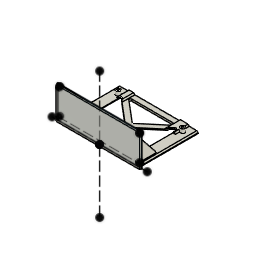
Mainboard Mount - Blank (Autodesk Fusion 360 design; units mm, degrees)
Autodesk Fusion 360 part; units mm, degrees
sketch "Sketch1" plane through (0, 0, 0) normal (0, 1, 0) x (1, 0, 0) in component "Blank Mount"
  line L0 (-75, 0) -> (75, 0) construction
  line L1 (-66, -50) -> (66, -50)
  line L2 (66, -50) -> (66, 0)
  line L3 (66, 0) -> (-66, 0)
  line L4 (-66, 0) -> (-66, -50)
  line L5 (0, -100) -> (0, 100) construction
  circle A0 centre (-63, -47) radius 1.75
  circle A1 centre (-63, -47) radius 3
  circle A2 centre (-63, -6.75) radius 1.75
  circle A3 centre (-63, -6.75) radius 3
  circle A4 centre (63, -47) radius 1.75
  circle A5 centre (63, -47) radius 3
  circle A6 centre (63, -6.75) radius 1.75
  circle A7 centre (63, -6.75) radius 3
  line L6 (-66, -5) -> (66, -5) construction
  dimension "d99_1" = 150
  dimension "d100_1" = 132
  dimension "d101_1" = 50
  dimension "d102_1" = 200
  dimension "d103_1" = 3.5
  dimension "d104_1" = 6
  dimension "d105_1" = 3.5
  dimension "d106_1" = 6
  dimension "d107_1" = 3.5
  dimension "d108_1" = 6
  dimension "d109_1" = 3.5
  dimension "d110_1" = 6
  dimension "d111_1" = 5
  constraint horizontal L0
  constraint midpoint L0 origin
  constraint horizontal L1
  constraint vertical L2
  constraint horizontal L3
  constraint vertical L4
  constraint vertical L5
  constraint midpoint L5 origin
  constraint midpoint L3 origin
  constraint coincident L5 origin
  constraint concentric A0 A1
  constraint concentric A2 A3
  constraint concentric A4 A5
  constraint concentric A6 A7
  constraint horizontal A0.centre A4.centre
  constraint vertical A4.centre A6.centre
  constraint vertical A0.centre A2.centre
  constraint horizontal A2.centre A6.centre
  constraint tangent L1 A1
  constraint tangent L4 A1
  constraint tangent L2 A5
  constraint coincident L4 L6.start
  constraint coincident L2 L6.end
  constraint perpendicular L2 L6
  constraint tangent A6 L6
  measures "d99_1" distance of L0.start L0.end
  measures "d100_1" distance of L1.start L1.end
  measures "d101_1" distance of L1.start L3.end
  measures "d102_1" distance of L5.start L5.end
  measures "d103_1" diameter of A0
  measures "d104_1" diameter of A1
  measures "d105_1" diameter of A2
  measures "d106_1" diameter of A3
  measures "d107_1" diameter of A4
  measures "d108_1" diameter of A5
  measures "d109_1" diameter of A6
  measures "d110_1" diameter of A7
  measures "d111_1" distance of L3 L6
extrude "Extrude1" add sketch "Sketch1" against normal blind 3 contours A7 | A3 | L1 L2 L3 L4 A1 A5 | A1 | A5 makes body 1 in component "Blank Mount"
sketch "Sketch2" plane through (0, 0, 0) normal (0, 1, 0) x (-1, 0, 0) in component "Blank Mount"
  circle A0 centre (-63, 6.75) radius 1.75
  circle A1 centre (-63, 47) radius 1.75
  circle A2 centre (63, 6.75) radius 1.75
  circle A3 centre (63, 47) radius 1.75
  line L0 (63, 50) -> (-63, 50)
  arc A4 (-63, 50) -> (-66, 47) centre (-63, 47) ccw
  line L1 (-66, 47) -> (-66, 0)
  line L2 (-66, 0) -> (66, 0)
  line L3 (66, 0) -> (66, 47)
  arc A5 (66, 47) -> (63, 50) centre (63, 47) ccw
  line L4 (-66, 3) -> (66, 3)
  line L5 (-62.8, 0) -> (-62.8, 1)
  line L6 (-62.8, 1) -> (-60.8, 3)
  line L7 (-62.8, 1) -> (-57.1716, 1) construction
  line L8 (62.8, 0) -> (62.8, 1)
  line L9 (62.8, 1) -> (60.8, 3)
  dimension "d114_1" = 3
  dimension "d115_1" = 1
  dimension "d116_1" = 45
  dimension "d117_1" = 3.2
  dimension "d118_1" = 1
  dimension "d119_1" = 135
  dimension "d121_1" = 125.6
  constraint coincident L1 L4.start
  constraint coincident L3 L4.end
  constraint perpendicular L3 L4
  constraint coincident L2 L5.start
  constraint perpendicular L2 L5
  constraint horizontal L7
  constraint coincident L4 L6.end
  constraint coincident L2 L8.start
  constraint perpendicular L2 L8
  constraint coincident L4 L9.end
  measures "d114_1" distance of L2 L4
  measures "d115_1" distance of L5.start L5.end
  measures "d116_1" angle of L6 L7
  measures "d117_1" distance of L1 L5
  measures "d118_1" distance of L8.start L8.end
  measures "d119_1" angle of L8 L9
  measures "d121_1" distance of L5.start L8.start
extrude "Extrude2" add sketch "Sketch2" along normal blind 92.3 contours L2 L4 L5 L6 L8 L9 bodies 1 in component "Blank Mount"
sketch "Sketch3" plane through (0, 0, 3) normal (0, 0, 1) x (-1, 0, 0) in component "Blank Mount"
  line L0 (60.8, 0) -> (-60.8, 0)
  line L1 (-60.8, 0) -> (-60.8, -92.3)
  line L2 (-60.8, -92.3) -> (60.8, -92.3)
  line L3 (60.8, -92.3) -> (60.8, 0)
  line L4 (0, 0) -> (0, -92.3) construction
  line L5 (62.8, 0, -3) -> (62.8, -92.3, -3) construction
  line L6 (62.8, -46.15, -3) -> (61.8909, -46.15, -3) construction
  line L7 (-62.8, 0, -2) -> (-62.8, -92.3, -2) construction
  line L8 (61.8909, -46.15, -3) -> (-62.8, -46.15, -2) construction
  circle A0 centre (51, -3.75) radius 1.45
  circle A1 centre (51, -3.75) radius 3.5
  circle A2 centre (51, -79.85) radius 1.45
  circle A3 centre (51, -79.85) radius 3.5
  circle A4 centre (-51, -3.75) radius 1.45
  circle A5 centre (-51, -3.75) radius 3.5
  circle A6 centre (-51, -79.85) radius 1.45
  circle A7 centre (-51, -79.85) radius 3.5
  line L9 (45, -84.15) -> (-45, -84.15)
  line L10 (-45, -84.15) -> (-45, -8.15)
  line L11 (-45, -8.15) -> (45, -8.15)
  line L12 (45, -8.15) -> (45, -84.15)
  line L13 (45, -8.15) -> (-45, -84.15) construction
  line L14 (45, -84.15) -> (-45, -8.15) construction
  line L15 (45, -78.9146) -> (6.1998, -46.15)
  line L16 (0, -40.9146) -> (-38.8002, -8.15)
  line L17 (38.8002, -84.15) -> (0, -51.3854)
  line L18 (-6.1998, -46.15) -> (-45, -13.3854)
  line L19 (45, -13.3854) -> (6.1998, -46.15)
  line L20 (0, -51.3854) -> (-38.8002, -84.15)
  line L21 (38.8002, -8.15) -> (0, -40.9146)
  line L22 (-6.1998, -46.15) -> (-45, -78.9146)
  point P0 (0, -46.15)
  dimension "d124_1" = 2.9
  dimension "d125_1" = 7
  dimension "d126_1" = 2.9
  dimension "d127_1" = 7
  dimension "d128_1" = 2.9
  dimension "d129_1" = 7
  dimension "d130_1" = 2.9
  dimension "d131_1" = 7
  dimension "d132_1" = 76.1
  dimension "d133_1" = 102
  dimension "d134_1" = 3.75
  dimension "d149_1" = 90
  dimension "d150_1" = 76
  dimension "d151_1" = 38
  dimension "d154_1" = 4
  dimension "d155_1" = 4
  constraint coincident L4.start origin
  constraint midpoint L2 L4.end
  constraint concentric A0 A1
  constraint concentric A2 A3
  constraint concentric A4 A5
  constraint concentric A6 A7
  constraint vertical A0.centre A2.centre
  constraint horizontal A0.centre A4.centre
  constraint horizontal A2.centre A6.centre
  constraint vertical A4.centre A6.centre
  constraint symmetric L4 A2.centre A6.centre
  constraint horizontal L9
  constraint vertical L10
  constraint horizontal L11
  constraint vertical L12
  constraint midpoint L4 P0
  constraint coincident L9 L17.start
  constraint coincident L10 L18.end
  constraint coincident L12 L15.start
  constraint coincident L11 L16.end
  constraint parallel L15 L17
  constraint coincident L12 L19.start
  constraint coincident L9 L20.end
  constraint coincident L11 L21.start
  constraint coincident L10 L22.end
  constraint parallel L19 L21
  constraint parallel L13 L21
  constraint parallel L14 L17
  constraint coincident L4 L16.start
  constraint collinear L15 L16
  constraint coincident L4 L17.end
  constraint collinear L17 L18
  constraint coincident L18.start L21
  constraint collinear L19 L20
  constraint collinear L21 L22
  measures "d124_1" diameter of A0
  measures "d125_1" diameter of A1
  measures "d126_1" diameter of A2
  measures "d127_1" diameter of A3
  measures "d128_1" diameter of A4
  measures "d129_1" diameter of A5
  measures "d130_1" diameter of A6
  measures "d131_1" diameter of A7
  measures "d132_1" distance of A0.centre A2.centre
  measures "d133_1" distance of A2.centre A6.centre
  measures "d134_1" distance of L0 A0.centre
  measures "d149_1" distance of L9.start L9.end
  measures "d150_1" distance of L9 L11
  measures "d151_1" distance of L9 P0
  measures "d154_1" distance of L13 L21
  measures "d155_1" distance of L14 L15
extrude "Extrude6" cut sketch "Sketch3" against normal blind 3 contours L9 L17 L20 | L12 L15 L19 | L10 L18 L22 | L11 L16 L21 bodies 1 in component "Blank Mount"
extrude "Extrude3" add sketch "Sketch3" along normal blind 6 contours A1 | A3 | A5 | A7 bodies 1 in component "Blank Mount"
fillet "Fillet1" radius 2 12 edges at (-38.8002, 84.15, 1.5) (6.1998, 46.15, 1.5) (0, 51.3854, 1.5) (-6.1998, 46.15, 1.5) (0, 40.9146, 1.5) (38.8002, 84.15, 1.5) (-45, 13.3854, 1.5) (-45, 78.9146, 1.5) (45, 78.9146, 1.5) (45, 13.3854, 1.5) (38.8002, 8.15, 1.5) (-38.8002, 8.15, 1.5) on bodies 1 in component "Blank Mount"
chamfer "Chamfer1" distance 5 angle 45 1 edges at (0, 0, 3) on bodies 1 in component "Blank Mount"
sketch "Sketch6" plane through (0, 0, 0) normal (0, 0, -1) x (1, 0, 0) in component "Blank Mount"
  line L0 (66, 3) -> (-66, 3)
  line L1 (62.8, 0) -> (66, 0)
  line L2 (-62.8, 0) -> (-62.8, -92.3)
  line L3 (-62.8, -92.3) -> (62.8, -92.3)
  line L4 (62.8, -92.3) -> (62.8, 0)
  line L5 (1.2904, -52.475) -> (34.6222, -80.6219)
  arc A0 (33.3319, -84.15) -> (34.6222, -80.6219) centre (33.3319, -82.15) ccw
  line L6 (33.3319, -84.15) -> (-33.3319, -84.15)
  arc A1 (-34.6222, -80.6219) -> (-33.3319, -84.15) centre (-33.3319, -82.15) ccw
  line L7 (-34.6222, -80.6219) -> (-1.2904, -52.475)
  arc A2 (1.2904, -52.475) -> (-1.2904, -52.475) centre (0, -54.0031) ccw
  line L8 (45, -17.692) -> (45, -74.608)
  arc A3 (41.7096, -76.1361) -> (45, -74.608) centre (43, -74.608) ccw
  line L9 (41.7096, -76.1361) -> (8.0094, -47.6781)
  arc A4 (8.0094, -44.6219) -> (8.0094, -47.6781) centre (9.2997, -46.15) ccw
  line L10 (8.0094, -44.6219) -> (41.7096, -16.1639)
  arc A5 (45, -17.692) -> (41.7096, -16.1639) centre (43, -17.692) ccw
  line L11 (-41.7096, -16.1639) -> (-8.0094, -44.6219)
  arc A6 (-8.0094, -47.6781) -> (-8.0094, -44.6219) centre (-9.2997, -46.15) ccw
  line L12 (-8.0094, -47.6781) -> (-41.7096, -76.1361)
  arc A7 (-45, -74.608) -> (-41.7096, -76.1361) centre (-43, -74.608) ccw
  line L13 (-45, -74.608) -> (-45, -17.692)
  arc A8 (-41.7096, -16.1639) -> (-45, -17.692) centre (-43, -17.692) ccw
  line L14 (34.6222, -11.6781) -> (1.2904, -39.825)
  arc A9 (-1.2904, -39.825) -> (1.2904, -39.825) centre (0, -38.2969) ccw
  line L15 (-1.2904, -39.825) -> (-34.6222, -11.6781)
  arc A10 (-33.3319, -8.15) -> (-34.6222, -11.6781) centre (-33.3319, -10.15) ccw
  line L16 (-33.3319, -8.15) -> (33.3319, -8.15)
  arc A11 (34.6222, -11.6781) -> (33.3319, -8.15) centre (33.3319, -10.15) ccw
  line L17 (41.3, -101.9006) -> (41.3, -57.1584) construction
  line L18 (37, -95.8656) -> (45, -95.8656)
  line L19 (45, -95.8656) -> (45, -65.8987)
  line L20 (45, -65.8987) -> (37, -65.8987)
  line L21 (37, -65.8987) -> (37, -95.8656)
  line L22 (66, 0) -> (66, 3)
  line L23 (-66, 3) -> (-66, 0)
  line L24 (-66, 0) -> (-62.8, 0)
  dimension "d215_1" = 21.5
  dimension "d216_1" = 8
  constraint vertical L17
  constraint horizontal L18
  constraint vertical L19
  constraint horizontal L20
  constraint vertical L21
  constraint collinear L8 L19
  measures "d215_1" distance of L4 L17
  measures "d216_1" distance of L18.start L18.end
extrude "Extrude8" cut sketch "Sketch6" against normal blind 2.9 contours L3 A3 L9 L19 L21 bodies 1 in component "Blank Mount"
sketch "Sketch7" plane through (0, 0, 3) normal (0, 0, 1) x (-1, 0, 0) in component "Blank Mount"
  circle A0 centre (-51, -79.85) radius 3.5
  line L0 (60.8, -5) -> (54.2692, -5)
  arc A1 (47.7308, -5) -> (54.2692, -5) centre (51, -3.75) ccw
  line L1 (47.7308, -5) -> (-47.7308, -5)
  arc A2 (-54.2692, -5) -> (-47.7308, -5) centre (-51, -3.75) ccw
  line L2 (-54.2692, -5) -> (-60.8, -5)
  line L3 (-60.8, -5) -> (-60.8, -92.3)
  line L4 (-60.8, -92.3) -> (60.8, -92.3)
  line L5 (60.8, -92.3) -> (60.8, -5)
  line L6 (-1.2904, -39.825) -> (-34.6222, -11.6781)
  arc A3 (-33.3319, -8.15) -> (-34.6222, -11.6781) centre (-33.3319, -10.15) ccw
  line L7 (-33.3319, -8.15) -> (33.3319, -8.15)
  arc A4 (34.6222, -11.6781) -> (33.3319, -8.15) centre (33.3319, -10.15) ccw
  line L8 (34.6222, -11.6781) -> (1.2904, -39.825)
  arc A5 (-1.2904, -39.825) -> (1.2904, -39.825) centre (0, -38.2969) ccw
  line L9 (8.0094, -44.6219) -> (41.7096, -16.1639)
  arc A6 (45, -17.692) -> (41.7096, -16.1639) centre (43, -17.692) ccw
  line L10 (45, -17.692) -> (45, -74.608)
  arc A7 (41.7096, -76.1361) -> (45, -74.608) centre (43, -74.608) ccw
  line L11 (41.7096, -76.1361) -> (8.0094, -47.6781)
  arc A8 (8.0094, -44.6219) -> (8.0094, -47.6781) centre (9.2997, -46.15) ccw
  line L12 (-45, -74.608) -> (-45, -17.692)
  arc A9 (-41.7096, -16.1639) -> (-45, -17.692) centre (-43, -17.692) ccw
  line L13 (-41.7096, -16.1639) -> (-8.0094, -44.6219)
  arc A10 (-8.0094, -47.6781) -> (-8.0094, -44.6219) centre (-9.2997, -46.15) ccw
  line L14 (-8.0094, -47.6781) -> (-41.7096, -76.1361)
  arc A11 (-45, -74.608) -> (-41.7096, -76.1361) centre (-43, -74.608) ccw
  line L15 (-34.6222, -80.6219) -> (-1.2904, -52.475)
  arc A12 (1.2904, -52.475) -> (-1.2904, -52.475) centre (0, -54.0031) ccw
  line L16 (1.2904, -52.475) -> (34.6222, -80.6219)
  arc A13 (33.3319, -84.15) -> (34.6222, -80.6219) centre (33.3319, -82.15) ccw
  line L17 (33.3319, -84.15) -> (-33.3319, -84.15)
  arc A14 (-34.6222, -80.6219) -> (-33.3319, -84.15) centre (-33.3319, -82.15) ccw
  circle A15 centre (51, -79.85) radius 3.5
  line L18 (-45, -74.608) -> (-45, -92.3)
  line L19 (-37, -92.3) -> (-37, -72.159)
  line L20 (-35, -92.3) -> (-35, -72.159)
  line L21 (-47, -74.608) -> (-47, -92.3)
  line L22 (-35, -72.159) -> (-35, -70.4702)
  line L23 (-47, -74.608) -> (-47, -70.4702)
  line L24 (-47, -70.4702) -> (-35, -70.4702)
  line L25 (43.4, -92.3) -> (43.4, -10.892) construction
  line L26 (62.8, 0) -> (62.8, -92.3)
  line L27 (45, -0.1179) -> (38.9, -0.1179)
  line L28 (38.9, -0.1179) -> (38.9, -92.3)
  line L29 (38.9, -92.3) -> (45, -92.3)
  line L30 (45, -92.3) -> (45, -0.1179)
  dimension "d219_1" = 2
  dimension "d220_1" = 2
  dimension "d344_1" = 19.4
  dimension "d372_1" = 4.5
  constraint coincident L14 L22.end
  constraint parallel L20 L22
  constraint parallel L12 L23
  constraint perpendicular L22 L24
  constraint coincident L4 L25.start
  constraint perpendicular L4 L25
  constraint horizontal L27
  constraint vertical L28
  constraint horizontal L29
  constraint vertical L30
  constraint coincident L4 L28.end
  constraint collinear L10 L30
  measures "d344_1" distance of L25 L26
  measures "d372_1" distance of L25.start L28.end
extrude "Extrude16" add sketch "Sketch7" along normal blind 2 contours L4 A7 L11 L28 L29 L30 | L1 L9 A6 L28 L30 | L1 L27 L28 L30 bodies 1 in component "Blank Mount"
extrude "Extrude9" add sketch "Sketch7" along normal blind 2 contours L4 L14 A14 L19 L20 L22 | L4 L14 A11 L18 L19 | L4 L12 L18 L21 L23 L24 bodies 1 in component "Blank Mount"
chamfer "Chamfer4" distance 2.8 angle 45 1 edges at (37, 82.2295, 0) on bodies 1 in component "Blank Mount"
chamfer "Chamfer5" distance 2 angle 45 3 edges at (35, 87.7767, 3) (35, 75.7584, 3) (47, 81.3851, 3) on bodies 1 in component "Blank Mount"
chamfer "Chamfer6" distance 1 angle 45 3 edges at (38.3548, 73.3031, 5) (43.8424, 76.422, 5) (45, 72.5391, 5) on bodies 1 in component "Blank Mount"
sketch "Sketch9" plane through (0, 0, 0) normal (0, 0, -1) x (1, 0, 0) in component "Blank Mount"
  line L0 (34.2, -92.3) -> (34.2, -83.9518)
  arc A0 (33.3319, -84.15) -> (34.2, -83.9518) centre (33.3319, -82.15) ccw
  line L1 (33.3319, -84.15) -> (-33.3319, -84.15)
  arc A1 (-34.6222, -80.6219) -> (-33.3319, -84.15) centre (-33.3319, -82.15) ccw
  line L2 (-34.6222, -80.6219) -> (-1.2904, -52.475)
  arc A2 (1.2904, -52.475) -> (-1.2904, -52.475) centre (0, -54.0031) ccw
  line L3 (1.2904, -52.475) -> (34.2, -80.2654)
  line L4 (34.2, -80.2654) -> (34.2, -69.7946)
  line L5 (34.2, -69.7946) -> (8.0094, -47.6781)
  arc A3 (8.0094, -44.6219) -> (8.0094, -47.6781) centre (9.2997, -46.15) ccw
  line L6 (8.0094, -44.6219) -> (41.7096, -16.1639)
  arc A4 (45, -17.692) -> (41.7096, -16.1639) centre (43, -17.692) ccw
  line L7 (45, -17.692) -> (45, -92.3)
  line L8 (45, -92.3) -> (62.8, -92.3)
  line L9 (62.8, -92.3) -> (62.8, 0)
  line L10 (62.8, 0) -> (66, 0)
  line L11 (66, 0) -> (66, 3)
  line L12 (66, 3) -> (-66, 3)
  line L13 (-66, 3) -> (-66, 0)
  line L14 (-66, 0) -> (-62.8, 0)
  line L15 (-62.8, 0) -> (-62.8, -92.3)
  line L16 (-41.7096, -16.1639) -> (-8.0094, -44.6219)
  arc A5 (-8.0094, -47.6781) -> (-8.0094, -44.6219) centre (-9.2997, -46.15) ccw
  line L17 (-8.0094, -47.6781) -> (-41.7096, -76.1361)
  arc A6 (-45, -74.608) -> (-41.7096, -76.1361) centre (-43, -74.608) ccw
  line L18 (-45, -74.608) -> (-45, -17.692)
  arc A7 (-41.7096, -16.1639) -> (-45, -17.692) centre (-43, -17.692) ccw
  line L19 (34.6222, -11.6781) -> (1.2904, -39.825)
  arc A8 (-1.2904, -39.825) -> (1.2904, -39.825) centre (0, -38.2969) ccw
  line L20 (-1.2904, -39.825) -> (-34.6222, -11.6781)
  arc A9 (-33.3319, -8.15) -> (-34.6222, -11.6781) centre (-33.3319, -10.15) ccw
  line L21 (-33.3319, -8.15) -> (33.3319, -8.15)
  arc A10 (34.6222, -11.6781) -> (33.3319, -8.15) centre (33.3319, -10.15) ccw
  line L22 (-45, -3) -> (-39.4, -3)
  line L23 (-39.4, -3) -> (-39.4, -74.1857)
  line L24 (-62.8, -92.3) -> (34.2, -92.3)
  line L25 (-45, -5) -> (-45, -17.692)
  line L26 (-45, -17.692) -> (-45, -74.608)
  line L27 (-45, -74.608) -> (-45, -92.3)
  line L28 (-45, -5) -> (-45, -3)
  line L29 (-39.4, -74.1857) -> (-39.4, -92.3079)
  constraint perpendicular L22 L23
  constraint coincident A6.start L18.start
  constraint coincident L24 L27.end
  constraint tangent A6 L27
  constraint coincident L25.start L28.start
  constraint coincident L22 L28.end
  constraint perpendicular L22 L28
  constraint vertical L29
extrude "Extrude13" cut sketch "Sketch9" against normal blind 2 contours L16 L17 A6 L18 A7 L23 L26 bodies 1 in component "Blank Mount"
sketch "Sketch10" plane through (0, 0, 3) normal (0, 0, 1) x (-1, 0, 0) in component "Blank Mount"
  arc A0 (-54.2692, -5) -> (-47.7308, -5) centre (-51, -3.75) ccw
  line L0 (-54.2692, -5) -> (-60.8, -5)
  line L1 (-60.8, -5) -> (-60.8, -92.3)
  line L2 (-33, -92.3) -> (38.9, -92.3)
  line L3 (-49, -92.3) -> (-49, -82.7223)
  arc A1 (-49, -76.9777) -> (-49, -82.7223) centre (-51, -79.85) ccw
  line L4 (-49, -76.9777) -> (-49, -70.4702)
  line L5 (-49, -70.4702) -> (-45, -70.4702)
  line L6 (-45, -70.4702) -> (-45, -17.692)
  arc A2 (-41.7096, -16.1639) -> (-45, -17.692) centre (-43, -17.692) ccw
  line L7 (-41.7096, -16.1639) -> (-8.0094, -44.6219)
  arc A3 (-8.0094, -47.6781) -> (-8.0094, -44.6219) centre (-9.2997, -46.15) ccw
  line L8 (-8.0094, -47.6781) -> (-33, -68.7813)
  line L9 (-33, -68.7813) -> (-33, -79.2521)
  line L10 (-33, -79.2521) -> (-1.2904, -52.475)
  arc A4 (1.2904, -52.475) -> (-1.2904, -52.475) centre (0, -54.0031) ccw
  line L11 (1.2904, -52.475) -> (34.6222, -80.6219)
  arc A5 (33.3319, -84.15) -> (34.6222, -80.6219) centre (33.3319, -82.15) ccw
  line L12 (33.3319, -84.15) -> (-33, -84.15)
  line L13 (-33, -84.15) -> (-33, -92.3)
  line L14 (38.9, -73.7635) -> (8.0094, -47.6781)
  arc A6 (8.0094, -44.6219) -> (8.0094, -47.6781) centre (9.2997, -46.15) ccw
  line L15 (8.0094, -44.6219) -> (38.9, -18.5365)
  line L16 (-1.2904, -39.825) -> (-34.6222, -11.6781)
  arc A7 (-33.3319, -8.15) -> (-34.6222, -11.6781) centre (-33.3319, -10.15) ccw
  line L17 (-33.3319, -8.15) -> (33.3319, -8.15)
  arc A8 (34.6222, -11.6781) -> (33.3319, -8.15) centre (33.3319, -10.15) ccw
  line L18 (34.6222, -11.6781) -> (1.2904, -39.825)
  arc A9 (-1.2904, -39.825) -> (1.2904, -39.825) centre (0, -38.2969) ccw
  line L19 (-56, -30) -> (-59, -30)
  line L20 (-59, -30) -> (-59, 0)
  line L21 (-59, 0) -> (-56, 0)
  line L22 (-56, 0) -> (-56, -30)
  line L23 (-85.9209, 0) -> (85.9209, 0) construction
  line L24 (38.9, -5) -> (-47.7308, -5)
  line L25 (38.9, -92.3) -> (38.9, -73.7635)
  line L26 (38.9, -18.5365) -> (38.9, -5)
  line L27 (-60.8, -92.3) -> (-49, -92.3)
  line L28 (45, -74.608) -> (45, -92.3)
  line L29 (56, 0) -> (59, 0)
  line L30 (59, 0) -> (59, -30)
  line L31 (59, -30) -> (56, -30)
  line L32 (56, -30) -> (56, 0)
  circle A10 centre (51, -3.75) radius 1.45
  circle A11 centre (51, -3.75) radius 3.5
  line L33 (60.8, -5) -> (60.8, -92.3)
  line L34 (47.0534, -7.25) -> (60.8, -7.25)
  dimension "d358_1" = 3
  dimension "d360_1" = 30
  dimension "d361_1" = 5
  dimension "d370_1" = 5
  dimension "d371_1" = 8
  dimension "d377_1" = 2
  dimension "d380_1" = 2
  dimension "d383_1" = 1.95
  dimension "d384_1" = 1.95
  dimension "d385_1" = 2
  dimension "d386_1" = 2
  dimension "d11" = 3
  dimension "d12" = 30
  dimension "d13" = 5
  constraint horizontal L19
  constraint vertical L20
  constraint horizontal L21
  constraint vertical L22
  constraint perpendicular L20 L23
  constraint midpoint origin L23
  constraint collinear L21 L23
  constraint horizontal L29
  constraint vertical L30
  constraint horizontal L31
  constraint vertical L32
  constraint coincident L23 L29.start
  constraint coincident L33 L34.end
  constraint perpendicular L30 L34
  constraint tangent A11 L34
  measures "d358_1" distance of L19.start L19.end
  measures "d360_1" distance of L19.end L20.end
  measures "d361_1" distance of A0.centre L22
  measures "d11" distance of L29.start L29.end
  measures "d12" distance of L29.start L31.end
  measures "d13" distance of L32 A10.centre
extrude "Extrude21" add sketch "Sketch10" along normal blind 36 contours L29 L30 L32 L34 bodies 1 in component "Blank Mount"
extrude "Extrude14" add sketch "Sketch10" along normal blind 36 contours L0 L19 L20 L22 | L0 L20 L21 L22 bodies 1 in component "Blank Mount"
chamfer "Chamfer9" distance 28 distance2 35 1 edges at (57.5, 30, 39) measured on face at (58, 10, 39) on bodies 1 in component "Blank Mount"
chamfer "Chamfer19" distance 2 angle 45 5 edges at (21.1047, 58.7363, 0) (7.2997, 46.15, 0) (24.8595, 30.3929, 0) (43.8424, 15.878, 0) (45, 54.996, 0) on bodies 1 in component "Blank Mount"
sketch "Sketch1 (2)" plane through (0, 0, 0) normal (0, 0, -1) x (1, 0, 0)
  line L0 (47, -17.692) -> (47, -92.3)
  line L1 (47, -92.3) -> (62.8, -92.3)
  line L2 (62.8, -92.3) -> (62.8, 0)
  line L3 (62.8, 0) -> (66, 0)
  line L4 (66, 0) -> (66, 3)
  line L5 (66, 3) -> (-66, 3)
  line L6 (-66, 3) -> (-66, 0)
  line L7 (-66, 0) -> (-62.8, 0)
  line L8 (-62.8, 0) -> (-62.8, -92.3)
  line L9 (-62.8, -92.3) -> (34.2, -92.3)
  line L10 (34.2, -92.3) -> (34.2, -83.9518)
  arc A0 (33.3319, -84.15) -> (34.2, -83.9518) centre (33.3319, -82.15) ccw
  line L11 (33.3319, -84.15) -> (-33.3319, -84.15)
  arc A1 (-34.6222, -80.6219) -> (-33.3319, -84.15) centre (-33.3319, -82.15) ccw
  line L12 (-34.6222, -80.6219) -> (-1.2904, -52.475)
  arc A2 (1.2904, -52.475) -> (-1.2904, -52.475) centre (0, -54.0031) ccw
  line L13 (1.2904, -52.475) -> (34.2, -80.2654)
  line L14 (34.2, -80.2654) -> (34.2, -72.4123)
  line L15 (34.2, -72.4123) -> (6.719, -49.2061)
  arc A3 (6.719, -43.0939) -> (6.719, -49.2061) centre (9.2997, -46.15) ccw
  line L16 (6.719, -43.0939) -> (40.4193, -14.6359)
  arc A4 (47, -17.692) -> (40.4193, -14.6359) centre (43, -17.692) ccw
  line L17 (-41.7096, -16.1639) -> (-8.0094, -44.6219)
  arc A5 (-8.0094, -47.6781) -> (-8.0094, -44.6219) centre (-9.2997, -46.15) ccw
  line L18 (-8.0094, -47.6781) -> (-41.7096, -76.1361)
  arc A6 (-45, -74.608) -> (-41.7096, -76.1361) centre (-43, -74.608) ccw
  line L19 (-45, -74.608) -> (-45, -17.692)
  arc A7 (-41.7096, -16.1639) -> (-45, -17.692) centre (-43, -17.692) ccw
  line L20 (34.6222, -11.6781) -> (1.2904, -39.825)
  arc A8 (-1.2904, -39.825) -> (1.2904, -39.825) centre (0, -38.2969) ccw
  line L21 (-1.2904, -39.825) -> (-34.6222, -11.6781)
  arc A9 (-33.3319, -8.15) -> (-34.6222, -11.6781) centre (-33.3319, -10.15) ccw
  line L22 (-33.3319, -8.15) -> (33.3319, -8.15)
  arc A10 (34.6222, -11.6781) -> (33.3319, -8.15) centre (33.3319, -10.15) ccw
  line L23 (-45, -74.608) -> (-45, -92.3)
  line L24 (-38.9, -92.3) -> (-38.9, -73.7635)
  line L25 (-45, -5) -> (-45, -17.692)
  line L26 (-38.9, -18.5365) -> (-38.9, -5)
  line L27 (-38.9, -3) -> (-45, -3)
  line L28 (-38.9, -92.3) -> (-45, -92.3)
  line L29 (-45, -92.3) -> (-45, -3)
  line L30 (-45, -3) -> (-38.9, -3)
  line L31 (-38.9, -3) -> (-38.9, -92.3)
  constraint horizontal L28
  constraint vertical L29
  constraint horizontal L30
  constraint vertical L31
  constraint coincident L27.end L29.end
  constraint coincident L24.start L28.start
extrude "Extrude19" cut sketch "Sketch1 (2)" against normal blind 2.9 contours L9 L18 A6 L23 L24 L28 L29 L31 | L17 A7 L25 L26 L27 L29 L30 L31 bodies 1 in component "Blank Mount"
chamfer "Chamfer20" distance 2 angle 45 1 edges at (-38.9, 83.0317, 3) on bodies 1 in component "Blank Mount"
chamfer "Chamfer21" distance 2 angle 45 1 edges at (-38.9, 11.7683, 3) on bodies 1 in component "Blank Mount"
extrude "Extrude20" add 2 faces at (-45, 8.564, 4.3333) (-45, 86.4027, 4.3333) along direction (-1, 0, 0) blind 1 on bodies 1 bodies 1 in component "Blank Mount"
chamfer "Chamfer22" distance 2 angle 45 2 edges at (-46, 83.454, 3) (-46, 11.346, 3) on bodies 1 in component "Blank Mount"
fillet "Fillet5" radius 1 6 edges at (-40.3048, 17.3502, 5) (-43.8424, 15.878, 5) (-45.5, 17.692, 5) (-43.8424, 76.422, 5) (-40.3048, 74.9498, 5) (-45.5, 74.608, 5) on bodies 1 in component "Blank Mount"
chamfer "Chamfer23" distance 2 angle 45 2 edges at (-38.9, 10.7683, 0) (-38.9, 83.0317, 0) on bodies 1 in component "Blank Mount"
chamfer "Chamfer24" distance 2 angle 45 1 edges at (-45, 47.65, 0) on bodies 1 in component "Blank Mount"
chamfer "Chamfer25" distance 5 angle 45 1 edges at (-57.5, 7.25, 39) on bodies 1 in component "Blank Mount"
chamfer "Chamfer26" distance 6 angle 45 1 edges at (-57.5, 7.25, 3) on bodies 1 in component "Blank Mount"
sketch "Sketch1 (3)" plane through (0, 0, 0) normal (0, 1, 0) x (1, 0, 0) in component "MKS Gen L Mount"
  line L0 (-75, 0) -> (75, 0) construction
  line L1 (-66, -50) -> (66, -50)
  line L2 (66, -50) -> (66, 0)
  line L3 (66, 0) -> (-66, 0)
  line L4 (-66, 0) -> (-66, -50)
  line L5 (0, -100) -> (0, 100) construction
  circle A0 centre (-63, -47) radius 1.75
  circle A1 centre (-63, -47) radius 3
  circle A2 centre (-63, -6.75) radius 1.75
  circle A3 centre (-63, -6.75) radius 3
  circle A4 centre (63, -47) radius 1.75
  circle A5 centre (63, -47) radius 3
  circle A6 centre (63, -6.75) radius 1.75
  circle A7 centre (63, -6.75) radius 3
  line L6 (-66, -5) -> (66, -5) construction
  dimension "d99_1_1" = 150
  dimension "d100_1_1" = 132
  dimension "d101_1_1" = 50
  dimension "d102_1_1" = 200
  dimension "d103_1_1" = 3.5
  dimension "d104_1_1" = 6
  dimension "d105_1_1" = 3.5
  dimension "d106_1_1" = 6
  dimension "d107_1_1" = 3.5
  dimension "d108_1_1" = 6
  dimension "d109_1_1" = 3.5
  dimension "d110_1_1" = 6
  dimension "d111_1_1" = 5
  constraint horizontal L0
  constraint midpoint L0 origin
  constraint horizontal L1
  constraint vertical L2
  constraint horizontal L3
  constraint vertical L4
  constraint vertical L5
  constraint midpoint L5 origin
  constraint midpoint L3 origin
  constraint coincident L5 origin
  constraint concentric A0 A1
  constraint concentric A2 A3
  constraint concentric A4 A5
  constraint concentric A6 A7
  constraint horizontal A0.centre A4.centre
  constraint vertical A4.centre A6.centre
  constraint vertical A0.centre A2.centre
  constraint horizontal A2.centre A6.centre
  constraint tangent L1 A1
  constraint tangent L4 A1
  constraint tangent L2 A5
  constraint coincident L4 L6.start
  constraint coincident L2 L6.end
  constraint perpendicular L2 L6
  constraint tangent A6 L6
  measures "d99_1_1" distance of L0.start L0.end
  measures "d100_1_1" distance of L1.start L1.end
  measures "d101_1_1" distance of L1.start L3.end
  measures "d102_1_1" distance of L5.start L5.end
  measures "d103_1_1" diameter of A0
  measures "d104_1_1" diameter of A1
  measures "d105_1_1" diameter of A2
  measures "d106_1_1" diameter of A3
  measures "d107_1_1" diameter of A4
  measures "d108_1_1" diameter of A5
  measures "d109_1_1" diameter of A6
  measures "d110_1_1" diameter of A7
  measures "d111_1_1" distance of L3 L6
extrude "Extrude1'" add sketch "Sketch1 (3)" against normal blind 3 separate body contours A7 | A3 | L1 L2 L3 L4 A1 A5 | A1 | A5 makes body 2 in component "MKS Gen L Mount"
sketch "Sketch2 (2)" plane through (0, 0, 0) normal (0, 1, 0) x (-1, 0, 0) in component "MKS Gen L Mount"
  circle A0 centre (-63, 6.75) radius 1.75
  circle A1 centre (-63, 47) radius 1.75
  circle A2 centre (63, 6.75) radius 1.75
  circle A3 centre (63, 47) radius 1.75
  line L0 (63, 50) -> (-63, 50)
  arc A4 (-63, 50) -> (-66, 47) centre (-63, 47) ccw
  line L1 (-66, 47) -> (-66, 0)
  line L2 (-66, 0) -> (66, 0)
  line L3 (66, 0) -> (66, 47)
  arc A5 (66, 47) -> (63, 50) centre (63, 47) ccw
  line L4 (-66, 3) -> (66, 3)
  line L5 (-62.8, 0) -> (-62.8, 1)
  line L6 (-62.8, 1) -> (-60.8, 3)
  line L7 (-62.8, 1) -> (-57.1716, 1) construction
  line L8 (62.8, 0) -> (62.8, 1)
  line L9 (62.8, 1) -> (60.8, 3)
  dimension "d114_1_1" = 3
  dimension "d115_1_1" = 1
  dimension "d116_1_1" = 45
  dimension "d117_1_1" = 3.2
  dimension "d118_1_1" = 1
  dimension "d119_1_1" = 135
  dimension "d121_1_1" = 125.6
  constraint coincident L1 L4.start
  constraint coincident L3 L4.end
  constraint perpendicular L3 L4
  constraint coincident L2 L5.start
  constraint perpendicular L2 L5
  constraint horizontal L7
  constraint coincident L4 L6.end
  constraint coincident L2 L8.start
  constraint perpendicular L2 L8
  constraint coincident L4 L9.end
  measures "d114_1_1" distance of L2 L4
  measures "d115_1_1" distance of L5.start L5.end
  measures "d116_1_1" angle of L6 L7
  measures "d117_1_1" distance of L1 L5
  measures "d118_1_1" distance of L8.start L8.end
  measures "d119_1_1" angle of L8 L9
  measures "d121_1_1" distance of L5.start L8.start
extrude "Extrude2'" add sketch "Sketch2 (2)" along normal blind 92.3 contours L2 L4 L5 L6 L8 L9 bodies 2 in component "MKS Gen L Mount"
sketch "Sketch3 (2)" plane through (0, 0, 3) normal (0, 0, 1) x (-1, 0, 0) in component "MKS Gen L Mount"
  line L0 (60.8, 0) -> (-60.8, 0)
  line L1 (-60.8, 0) -> (-60.8, -92.3)
  line L2 (-60.8, -92.3) -> (60.8, -92.3)
  line L3 (60.8, -92.3) -> (60.8, 0)
  line L4 (0, 0) -> (0, -92.3) construction
  line L5 (62.8, 0, -3) -> (62.8, -92.3, -3) construction
  line L6 (62.8, -46.15, -3) -> (61.8909, -46.15, -3) construction
  line L7 (-62.8, 0, -2) -> (-62.8, -92.3, -2) construction
  line L8 (61.8909, -46.15, -3) -> (-62.8, -46.15, -2) construction
  circle A0 centre (51, -3.75) radius 1.45
  circle A1 centre (51, -3.75) radius 3.5
  circle A2 centre (51, -79.85) radius 1.45
  circle A3 centre (51, -79.85) radius 3.5
  circle A4 centre (-51, -3.75) radius 1.45
  circle A5 centre (-51, -3.75) radius 3.5
  circle A6 centre (-51, -79.85) radius 1.45
  circle A7 centre (-51, -79.85) radius 3.5
  line L9 (45, -84.15) -> (-45, -84.15)
  line L10 (-45, -84.15) -> (-45, -8.15)
  line L11 (-45, -8.15) -> (45, -8.15)
  line L12 (45, -8.15) -> (45, -84.15)
  line L13 (45, -8.15) -> (-45, -84.15) construction
  line L14 (45, -84.15) -> (-45, -8.15) construction
  line L15 (45, -78.9146) -> (6.1998, -46.15)
  line L16 (0, -40.9146) -> (-38.8002, -8.15)
  line L17 (38.8002, -84.15) -> (0, -51.3854)
  line L18 (-6.1998, -46.15) -> (-45, -13.3854)
  line L19 (45, -13.3854) -> (6.1998, -46.15)
  line L20 (0, -51.3854) -> (-38.8002, -84.15)
  line L21 (38.8002, -8.15) -> (0, -40.9146)
  line L22 (-6.1998, -46.15) -> (-45, -78.9146)
  point P0 (0, -46.15)
  dimension "d124_1_1" = 2.9
  dimension "d125_1_1" = 7
  dimension "d126_1_1" = 2.9
  dimension "d127_1_1" = 7
  dimension "d128_1_1" = 2.9
  dimension "d129_1_1" = 7
  dimension "d130_1_1" = 2.9
  dimension "d131_1_1" = 7
  dimension "d132_1_1" = 76.1
  dimension "d133_1_1" = 102
  dimension "d134_1_1" = 3.75
  dimension "d149_1_1" = 90
  dimension "d150_1_1" = 76
  dimension "d151_1_1" = 38
  dimension "d154_1_1" = 4
  dimension "d155_1_1" = 4
  constraint coincident L4.start origin
  constraint midpoint L2 L4.end
  constraint concentric A0 A1
  constraint concentric A2 A3
  constraint concentric A4 A5
  constraint concentric A6 A7
  constraint vertical A0.centre A2.centre
  constraint horizontal A0.centre A4.centre
  constraint horizontal A2.centre A6.centre
  constraint vertical A4.centre A6.centre
  constraint symmetric L4 A2.centre A6.centre
  constraint horizontal L9
  constraint vertical L10
  constraint horizontal L11
  constraint vertical L12
  constraint midpoint L4 P0
  constraint coincident L9 L17.start
  constraint coincident L10 L18.end
  constraint coincident L12 L15.start
  constraint coincident L11 L16.end
  constraint parallel L15 L17
  constraint coincident L12 L19.start
  constraint coincident L9 L20.end
  constraint coincident L11 L21.start
  constraint coincident L10 L22.end
  constraint parallel L19 L21
  constraint parallel L13 L21
  constraint parallel L14 L17
  constraint coincident L4 L16.start
  constraint collinear L15 L16
  constraint coincident L4 L17.end
  constraint collinear L17 L18
  constraint coincident L18.start L21
  constraint collinear L19 L20
  constraint collinear L21 L22
  measures "d124_1_1" diameter of A0
  measures "d125_1_1" diameter of A1
  measures "d126_1_1" diameter of A2
  measures "d127_1_1" diameter of A3
  measures "d128_1_1" diameter of A4
  measures "d129_1_1" diameter of A5
  measures "d130_1_1" diameter of A6
  measures "d131_1_1" diameter of A7
  measures "d132_1_1" distance of A0.centre A2.centre
  measures "d133_1_1" distance of A2.centre A6.centre
  measures "d134_1_1" distance of L0 A0.centre
  measures "d149_1_1" distance of L9.start L9.end
  measures "d150_1_1" distance of L9 L11
  measures "d151_1_1" distance of L9 P0
  measures "d154_1_1" distance of L13 L21
  measures "d155_1_1" distance of L14 L15
extrude "Extrude6'" cut sketch "Sketch3 (2)" against normal blind 3 contours L9 L17 L20 | L12 L15 L19 | L10 L18 L22 | L11 L16 L21 bodies 2 in component "MKS Gen L Mount"
extrude "Extrude3'" add sketch "Sketch3 (2)" along normal blind 6 contours A1 | A3 | A5 | A7 bodies 2 in component "MKS Gen L Mount"
fillet "Fillet1'" radius 2 12 edges at (-38.8002, 84.15, 1.5) (6.1998, 46.15, 1.5) (0, 51.3854, 1.5) (-6.1998, 46.15, 1.5) (0, 40.9146, 1.5) (38.8002, 84.15, 1.5) (-45, 13.3854, 1.5) (-45, 78.9146, 1.5) (45, 78.9146, 1.5) (45, 13.3854, 1.5) (38.8002, 8.15, 1.5) (-38.8002, 8.15, 1.5) on bodies 2 in component "MKS Gen L Mount"
chamfer "Chamfer1'" distance 5 angle 45 1 edges at (0, 0, 3) on bodies 2 in component "MKS Gen L Mount"
sketch "Sketch6 (2)" plane through (0, 0, 0) normal (0, 0, -1) x (1, 0, 0) in component "MKS Gen L Mount"
  line L0 (66, 3) -> (-66, 3)
  line L1 (62.8, 0) -> (66, 0)
  line L2 (-62.8, 0) -> (-62.8, -92.3)
  line L3 (-62.8, -92.3) -> (62.8, -92.3)
  line L4 (62.8, -92.3) -> (62.8, 0)
  line L5 (1.2904, -52.475) -> (34.6222, -80.6219)
  arc A0 (33.3319, -84.15) -> (34.6222, -80.6219) centre (33.3319, -82.15) ccw
  line L6 (33.3319, -84.15) -> (-33.3319, -84.15)
  arc A1 (-34.6222, -80.6219) -> (-33.3319, -84.15) centre (-33.3319, -82.15) ccw
  line L7 (-34.6222, -80.6219) -> (-1.2904, -52.475)
  arc A2 (1.2904, -52.475) -> (-1.2904, -52.475) centre (0, -54.0031) ccw
  line L8 (45, -17.692) -> (45, -74.608)
  arc A3 (41.7096, -76.1361) -> (45, -74.608) centre (43, -74.608) ccw
  line L9 (41.7096, -76.1361) -> (8.0094, -47.6781)
  arc A4 (8.0094, -44.6219) -> (8.0094, -47.6781) centre (9.2997, -46.15) ccw
  line L10 (8.0094, -44.6219) -> (41.7096, -16.1639)
  arc A5 (45, -17.692) -> (41.7096, -16.1639) centre (43, -17.692) ccw
  line L11 (-41.7096, -16.1639) -> (-8.0094, -44.6219)
  arc A6 (-8.0094, -47.6781) -> (-8.0094, -44.6219) centre (-9.2997, -46.15) ccw
  line L12 (-8.0094, -47.6781) -> (-41.7096, -76.1361)
  arc A7 (-45, -74.608) -> (-41.7096, -76.1361) centre (-43, -74.608) ccw
  line L13 (-45, -74.608) -> (-45, -17.692)
  arc A8 (-41.7096, -16.1639) -> (-45, -17.692) centre (-43, -17.692) ccw
  line L14 (34.6222, -11.6781) -> (1.2904, -39.825)
  arc A9 (-1.2904, -39.825) -> (1.2904, -39.825) centre (0, -38.2969) ccw
  line L15 (-1.2904, -39.825) -> (-34.6222, -11.6781)
  arc A10 (-33.3319, -8.15) -> (-34.6222, -11.6781) centre (-33.3319, -10.15) ccw
  line L16 (-33.3319, -8.15) -> (33.3319, -8.15)
  arc A11 (34.6222, -11.6781) -> (33.3319, -8.15) centre (33.3319, -10.15) ccw
  line L17 (41.3, -101.9006) -> (41.3, -57.1584) construction
  line L18 (37, -95.8656) -> (45, -95.8656)
  line L19 (45, -95.8656) -> (45, -65.8987)
  line L20 (45, -65.8987) -> (37, -65.8987)
  line L21 (37, -65.8987) -> (37, -95.8656)
  line L22 (66, 0) -> (66, 3)
  line L23 (-66, 3) -> (-66, 0)
  line L24 (-66, 0) -> (-62.8, 0)
  dimension "d215_1_1" = 21.5
  dimension "d216_1_1" = 8
  constraint vertical L17
  constraint horizontal L18
  constraint vertical L19
  constraint horizontal L20
  constraint vertical L21
  constraint collinear L8 L19
  measures "d215_1_1" distance of L4 L17
  measures "d216_1_1" distance of L18.start L18.end
extrude "Extrude8'" cut sketch "Sketch6 (2)" against normal blind 2.9 contours L3 A3 L9 L19 L21 bodies 2 in component "MKS Gen L Mount"
sketch "Sketch7 (2)" plane through (0, 0, 3) normal (0, 0, 1) x (-1, 0, 0) in component "MKS Gen L Mount"
  circle A0 centre (-51, -79.85) radius 3.5
  line L0 (60.8, -5) -> (54.2692, -5)
  arc A1 (47.7308, -5) -> (54.2692, -5) centre (51, -3.75) ccw
  line L1 (47.7308, -5) -> (-47.7308, -5)
  arc A2 (-54.2692, -5) -> (-47.7308, -5) centre (-51, -3.75) ccw
  line L2 (-54.2692, -5) -> (-60.8, -5)
  line L3 (-60.8, -5) -> (-60.8, -92.3)
  line L4 (-60.8, -92.3) -> (60.8, -92.3)
  line L5 (60.8, -92.3) -> (60.8, -5)
  line L6 (-1.2904, -39.825) -> (-34.6222, -11.6781)
  arc A3 (-33.3319, -8.15) -> (-34.6222, -11.6781) centre (-33.3319, -10.15) ccw
  line L7 (-33.3319, -8.15) -> (33.3319, -8.15)
  arc A4 (34.6222, -11.6781) -> (33.3319, -8.15) centre (33.3319, -10.15) ccw
  line L8 (34.6222, -11.6781) -> (1.2904, -39.825)
  arc A5 (-1.2904, -39.825) -> (1.2904, -39.825) centre (0, -38.2969) ccw
  line L9 (8.0094, -44.6219) -> (41.7096, -16.1639)
  arc A6 (45, -17.692) -> (41.7096, -16.1639) centre (43, -17.692) ccw
  line L10 (45, -17.692) -> (45, -74.608)
  arc A7 (41.7096, -76.1361) -> (45, -74.608) centre (43, -74.608) ccw
  line L11 (41.7096, -76.1361) -> (8.0094, -47.6781)
  arc A8 (8.0094, -44.6219) -> (8.0094, -47.6781) centre (9.2997, -46.15) ccw
  line L12 (-45, -74.608) -> (-45, -17.692)
  arc A9 (-41.7096, -16.1639) -> (-45, -17.692) centre (-43, -17.692) ccw
  line L13 (-41.7096, -16.1639) -> (-8.0094, -44.6219)
  arc A10 (-8.0094, -47.6781) -> (-8.0094, -44.6219) centre (-9.2997, -46.15) ccw
  line L14 (-8.0094, -47.6781) -> (-41.7096, -76.1361)
  arc A11 (-45, -74.608) -> (-41.7096, -76.1361) centre (-43, -74.608) ccw
  line L15 (-34.6222, -80.6219) -> (-1.2904, -52.475)
  arc A12 (1.2904, -52.475) -> (-1.2904, -52.475) centre (0, -54.0031) ccw
  line L16 (1.2904, -52.475) -> (34.6222, -80.6219)
  arc A13 (33.3319, -84.15) -> (34.6222, -80.6219) centre (33.3319, -82.15) ccw
  line L17 (33.3319, -84.15) -> (-33.3319, -84.15)
  arc A14 (-34.6222, -80.6219) -> (-33.3319, -84.15) centre (-33.3319, -82.15) ccw
  circle A15 centre (51, -79.85) radius 3.5
  line L18 (-45, -74.608) -> (-45, -92.3)
  line L19 (-37, -92.3) -> (-37, -72.159)
  line L20 (-35, -92.3) -> (-35, -72.159)
  line L21 (-47, -74.608) -> (-47, -92.3)
  line L22 (-35, -72.159) -> (-35, -70.4702)
  line L23 (-47, -74.608) -> (-47, -70.4702)
  line L24 (-47, -70.4702) -> (-35, -70.4702)
  line L25 (43.4, -92.3) -> (43.4, -10.892) construction
  line L26 (62.8, 0) -> (62.8, -92.3)
  line L27 (45, -0.1179) -> (38.9, -0.1179)
  line L28 (38.9, -0.1179) -> (38.9, -92.3)
  line L29 (38.9, -92.3) -> (45, -92.3)
  line L30 (45, -92.3) -> (45, -0.1179)
  dimension "d219_1_1" = 2
  dimension "d220_1_1" = 2
  dimension "d344_1_1" = 19.4
  dimension "d372_1_1" = 4.5
  constraint coincident L14 L22.end
  constraint parallel L20 L22
  constraint parallel L12 L23
  constraint perpendicular L22 L24
  constraint coincident L4 L25.start
  constraint perpendicular L4 L25
  constraint horizontal L27
  constraint vertical L28
  constraint horizontal L29
  constraint vertical L30
  constraint coincident L4 L28.end
  constraint collinear L10 L30
  measures "d344_1_1" distance of L25 L26
  measures "d372_1_1" distance of L25.start L28.end
extrude "Extrude16'" add sketch "Sketch7 (2)" along normal blind 2 contours L4 A7 L11 L28 L29 L30 | L1 L9 A6 L28 L30 | L1 L27 L28 L30 bodies 2 in component "MKS Gen L Mount"
extrude "Extrude9'" add sketch "Sketch7 (2)" along normal blind 2 contours L4 L14 A14 L19 L20 L22 | L4 L14 A11 L18 L19 | L4 L12 L18 L21 L23 L24 bodies 2 in component "MKS Gen L Mount"
chamfer "Chamfer4'" distance 2.8 angle 45 1 edges at (37, 82.2295, 0) on bodies 2 in component "MKS Gen L Mount"
chamfer "Chamfer5'" distance 2 angle 45 3 edges at (35, 87.7767, 3) (35, 75.7584, 3) (47, 81.3851, 3) on bodies 2 in component "MKS Gen L Mount"
chamfer "Chamfer6'" distance 1 angle 45 3 edges at (38.3548, 73.3031, 5) (43.8424, 76.422, 5) (45, 72.5391, 5) on bodies 2 in component "MKS Gen L Mount"
sketch "Sketch9 (2)" plane through (0, 0, 0) normal (0, 0, -1) x (1, 0, 0) in component "MKS Gen L Mount"
  line L0 (34.2, -92.3) -> (34.2, -83.9518)
  arc A0 (33.3319, -84.15) -> (34.2, -83.9518) centre (33.3319, -82.15) ccw
  line L1 (33.3319, -84.15) -> (-33.3319, -84.15)
  arc A1 (-34.6222, -80.6219) -> (-33.3319, -84.15) centre (-33.3319, -82.15) ccw
  line L2 (-34.6222, -80.6219) -> (-1.2904, -52.475)
  arc A2 (1.2904, -52.475) -> (-1.2904, -52.475) centre (0, -54.0031) ccw
  line L3 (1.2904, -52.475) -> (34.2, -80.2654)
  line L4 (34.2, -80.2654) -> (34.2, -69.7946)
  line L5 (34.2, -69.7946) -> (8.0094, -47.6781)
  arc A3 (8.0094, -44.6219) -> (8.0094, -47.6781) centre (9.2997, -46.15) ccw
  line L6 (8.0094, -44.6219) -> (41.7096, -16.1639)
  arc A4 (45, -17.692) -> (41.7096, -16.1639) centre (43, -17.692) ccw
  line L7 (45, -17.692) -> (45, -92.3)
  line L8 (45, -92.3) -> (62.8, -92.3)
  line L9 (62.8, -92.3) -> (62.8, 0)
  line L10 (62.8, 0) -> (66, 0)
  line L11 (66, 0) -> (66, 3)
  line L12 (66, 3) -> (-66, 3)
  line L13 (-66, 3) -> (-66, 0)
  line L14 (-66, 0) -> (-62.8, 0)
  line L15 (-62.8, 0) -> (-62.8, -92.3)
  line L16 (-41.7096, -16.1639) -> (-8.0094, -44.6219)
  arc A5 (-8.0094, -47.6781) -> (-8.0094, -44.6219) centre (-9.2997, -46.15) ccw
  line L17 (-8.0094, -47.6781) -> (-41.7096, -76.1361)
  arc A6 (-45, -74.608) -> (-41.7096, -76.1361) centre (-43, -74.608) ccw
  line L18 (-45, -74.608) -> (-45, -17.692)
  arc A7 (-41.7096, -16.1639) -> (-45, -17.692) centre (-43, -17.692) ccw
  line L19 (34.6222, -11.6781) -> (1.2904, -39.825)
  arc A8 (-1.2904, -39.825) -> (1.2904, -39.825) centre (0, -38.2969) ccw
  line L20 (-1.2904, -39.825) -> (-34.6222, -11.6781)
  arc A9 (-33.3319, -8.15) -> (-34.6222, -11.6781) centre (-33.3319, -10.15) ccw
  line L21 (-33.3319, -8.15) -> (33.3319, -8.15)
  arc A10 (34.6222, -11.6781) -> (33.3319, -8.15) centre (33.3319, -10.15) ccw
  line L22 (-45, -3) -> (-39.4, -3)
  line L23 (-39.4, -3) -> (-39.4, -74.1857)
  line L24 (-62.8, -92.3) -> (34.2, -92.3)
  line L25 (-45, -5) -> (-45, -17.692)
  line L26 (-45, -17.692) -> (-45, -74.608)
  line L27 (-45, -74.608) -> (-45, -92.3)
  line L28 (-45, -5) -> (-45, -3)
  line L29 (-39.4, -74.1857) -> (-39.4, -92.3079)
  constraint perpendicular L22 L23
  constraint coincident A6.start L18.start
  constraint coincident L24 L27.end
  constraint tangent A6 L27
  constraint coincident L25.start L28.start
  constraint coincident L22 L28.end
  constraint perpendicular L22 L28
  constraint vertical L29
extrude "Extrude13'" cut sketch "Sketch9 (2)" against normal blind 2 contours L16 L17 A6 L18 A7 L23 L26 bodies 2 in component "MKS Gen L Mount"
sketch "Sketch10 (2)" plane through (0, 0, 3) normal (0, 0, 1) x (-1, 0, 0) in component "MKS Gen L Mount"
  arc A0 (-54.2692, -5) -> (-47.7308, -5) centre (-51, -3.75) ccw
  line L0 (-54.2692, -5) -> (-60.8, -5)
  line L1 (-60.8, -5) -> (-60.8, -92.3)
  line L2 (-33, -92.3) -> (38.9, -92.3)
  line L3 (-49, -92.3) -> (-49, -82.7223)
  arc A1 (-49, -76.9777) -> (-49, -82.7223) centre (-51, -79.85) ccw
  line L4 (-49, -76.9777) -> (-49, -70.4702)
  line L5 (-49, -70.4702) -> (-45, -70.4702)
  line L6 (-45, -70.4702) -> (-45, -17.692)
  arc A2 (-41.7096, -16.1639) -> (-45, -17.692) centre (-43, -17.692) ccw
  line L7 (-41.7096, -16.1639) -> (-8.0094, -44.6219)
  arc A3 (-8.0094, -47.6781) -> (-8.0094, -44.6219) centre (-9.2997, -46.15) ccw
  line L8 (-8.0094, -47.6781) -> (-33, -68.7813)
  line L9 (-33, -68.7813) -> (-33, -79.2521)
  line L10 (-33, -79.2521) -> (-1.2904, -52.475)
  arc A4 (1.2904, -52.475) -> (-1.2904, -52.475) centre (0, -54.0031) ccw
  line L11 (1.2904, -52.475) -> (34.6222, -80.6219)
  arc A5 (33.3319, -84.15) -> (34.6222, -80.6219) centre (33.3319, -82.15) ccw
  line L12 (33.3319, -84.15) -> (-33, -84.15)
  line L13 (-33, -84.15) -> (-33, -92.3)
  line L14 (38.9, -73.7635) -> (8.0094, -47.6781)
  arc A6 (8.0094, -44.6219) -> (8.0094, -47.6781) centre (9.2997, -46.15) ccw
  line L15 (8.0094, -44.6219) -> (38.9, -18.5365)
  line L16 (-1.2904, -39.825) -> (-34.6222, -11.6781)
  arc A7 (-33.3319, -8.15) -> (-34.6222, -11.6781) centre (-33.3319, -10.15) ccw
  line L17 (-33.3319, -8.15) -> (33.3319, -8.15)
  arc A8 (34.6222, -11.6781) -> (33.3319, -8.15) centre (33.3319, -10.15) ccw
  line L18 (34.6222, -11.6781) -> (1.2904, -39.825)
  arc A9 (-1.2904, -39.825) -> (1.2904, -39.825) centre (0, -38.2969) ccw
  line L19 (-56, -30) -> (-59, -30)
  line L20 (-59, -30) -> (-59, 0)
  line L21 (-59, 0) -> (-56, 0)
  line L22 (-56, 0) -> (-56, -30)
  line L23 (-85.9209, 0) -> (85.9209, 0) construction
  line L24 (38.9, -5) -> (-47.7308, -5)
  line L25 (38.9, -92.3) -> (38.9, -73.7635)
  line L26 (38.9, -18.5365) -> (38.9, -5)
  line L27 (-60.8, -92.3) -> (-49, -92.3)
  line L28 (45, -74.608) -> (45, -92.3)
  line L29 (56, 0) -> (59, 0)
  line L30 (59, 0) -> (59, -30)
  line L31 (59, -30) -> (56, -30)
  line L32 (56, -30) -> (56, 0)
  circle A10 centre (51, -3.75) radius 1.45
  circle A11 centre (51, -3.75) radius 3.5
  line L33 (60.8, -5) -> (60.8, -92.3)
  line L34 (47.0534, -7.25) -> (60.8, -7.25)
  dimension "d358_1_1" = 3
  dimension "d360_1_1" = 30
  dimension "d361_1_1" = 5
  dimension "d11_1" = 3
  dimension "d12_1" = 30
  dimension "d13_1" = 5
  constraint horizontal L19
  constraint vertical L20
  constraint horizontal L21
  constraint vertical L22
  constraint perpendicular L20 L23
  constraint midpoint origin L23
  constraint collinear L21 L23
  constraint horizontal L29
  constraint vertical L30
  constraint horizontal L31
  constraint vertical L32
  constraint coincident L23 L29.start
  constraint coincident L33 L34.end
  constraint perpendicular L30 L34
  constraint tangent A11 L34
  measures "d358_1_1" distance of L19.start L19.end
  measures "d360_1_1" distance of L19.end L20.end
  measures "d361_1_1" distance of A0.centre L22
  measures "d11_1" distance of L29.start L29.end
  measures "d12_1" distance of L29.start L31.end
  measures "d13_1" distance of L32 A10.centre
extrude "Extrude21'" add sketch "Sketch10 (2)" along normal blind 36 contours L29 L30 L32 L34 bodies 2 in component "MKS Gen L Mount"
extrude "Extrude14'" add sketch "Sketch10 (2)" along normal blind 36 contours L0 L19 L20 L22 | L0 L20 L21 L22 bodies 2 in component "MKS Gen L Mount"
chamfer "Chamfer9'" distance 28 distance2 35 1 edges at (57.5, 30, 39) measured on face at (58, 10, 39) on bodies 2 in component "MKS Gen L Mount"
chamfer "Chamfer19'" distance 2 angle 45 5 edges at (21.1047, 58.7363, 0) (7.2997, 46.15, 0) (24.8595, 30.3929, 0) (43.8424, 15.878, 0) (45, 54.996, 0) on bodies 2 in component "MKS Gen L Mount"
extrude "Extrude19'" cut sketch "Sketch1 (2)" against normal blind 2.9 contours L9 L18 A6 L23 L24 L28 L29 L31 | L17 A7 L25 L26 L27 L29 L30 L31 bodies 2 in component "MKS Gen L Mount"
chamfer "Chamfer20'" distance 2 angle 45 1 edges at (-38.9, 83.0317, 3) on bodies 2 in component "MKS Gen L Mount"
chamfer "Chamfer21'" distance 2 angle 45 1 edges at (-38.9, 11.7683, 3) on bodies 2 in component "MKS Gen L Mount"
extrude "Extrude20'" add 2 faces at (-45, 8.564, 4.3333) (-45, 86.4027, 4.3333) along direction (-1, 0, 0) blind 1 on bodies 2 bodies 2 in component "MKS Gen L Mount"
chamfer "Chamfer22'" distance 2 angle 45 2 edges at (-46, 83.454, 3) (-46, 11.346, 3) on bodies 2 in component "MKS Gen L Mount"
fillet "Fillet5'" radius 1 6 edges at (-40.3048, 17.3502, 5) (-43.8424, 15.878, 5) (-45.5, 17.692, 5) (-43.8424, 76.422, 5) (-40.3048, 74.9498, 5) (-45.5, 74.608, 5) on bodies 2 in component "MKS Gen L Mount"
chamfer "Chamfer23'" distance 2 angle 45 2 edges at (-38.9, 10.7683, 0) (-38.9, 83.0317, 0) on bodies 2 in component "MKS Gen L Mount"
chamfer "Chamfer24'" distance 2 angle 45 1 edges at (-45, 47.65, 0) on bodies 2 in component "MKS Gen L Mount"
chamfer "Chamfer25'" distance 5 angle 45 1 edges at (-57.5, 7.25, 39) on bodies 2 in component "MKS Gen L Mount"
chamfer "Chamfer26'" distance 6 angle 45 1 edges at (-57.5, 7.25, 3) on bodies 2 in component "MKS Gen L Mount"
component "Blank Mount" placed x (1, 0, 0) y (0, 1, 0) z (0, 0, 1) at (0, 0, 0)
component "MKS Gen L Mount" placed x (1, 0, 0) y (0, 1, 0) z (0, 0, 1) at (0, 0, 0)
equation "d117_1 = ( 132 mm - d121_1 ) / 2"
equation "d147_1 = 0.0 deg"
equation "d151_1 = d150_1 / 2"
equation "d155_1 = d154_1"
equation "d181_1 = 38.44 mm - 0.5 mm"
equation "d337_1 = 0.0 deg"
equation "d369_1 = 0.0 deg"
equation "d376_1 = 0.0 deg"
equation "d379_1 = 0.0 deg"
equation "d117_1_1 = ( 132 mm - d121_1_1 ) / 2"
equation "d151_1_1 = d150_1_1 / 2"
equation "d155_1_1 = d154_1_1"
